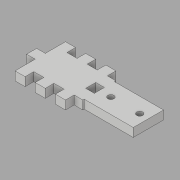
# Autodesk Inventor part: g_arm_v_1
Saved by Autodesk Inventor 2019 (Build 230136000, 136)
## iProperties
Created: 2021-11-02
Part Number: g_arm_v_1
Material: Generic
Document SubType Name: Modeling
Designer: Mohamed
Density: 1 g/cm^3
Appearance: Default
Author: Mohamed
Autodesk Inventor part; units mm, degrees
ref_plane "YZ Plane" through (0, 0, 0) normal (1, 0, 0) x (0, 1, 0)
ref_plane "XZ Plane" through (0, 0, 0) normal (0, 1, 0) x (-1, 0, 0)
ref_plane "XY Plane" through (0, 0, 0) normal (0, 0, 1) x (1, 0, 0)
sketch "Sketch1" plane through (0, 0, 0) normal (1, 0, 0) x (0, 1, 0)
  point P0 (0, 0)
sketch "Sketch2" plane through (0, 0, 0) normal (0, 1, 0) x (-1, 0, 0)
  line L0 (0, 0) -> (35, 0)
  line L1 (35, -21) -> (0, -21)
  line L2 (35, -7) -> (41, -7)
  line L3 (41, -7) -> (41, -14)
  line L4 (41, -14) -> (35, -14)
  line L5 (35, 0) -> (35, -7)
  line L6 (35, -14) -> (35, -21)
  line L7 (0, -21) -> (-40, -21)
  line L8 (-40, -21) -> (-40, 0)
  line L9 (-40, 0) -> (0, 0)
  circle A0 centre (-34, -10.5) radius 2.1
  circle A1 centre (-14, -10.5) radius 2.1
  line L10 (0, -7) -> (-6, -7)
  line L11 (-6, -7) -> (-6, -14)
  line L12 (-6, -14) -> (0, -14)
  line L13 (0, -14) -> (0, -7)
  dimension "d0" = 35
  dimension "d1" = 21
  dimension "d2" = 7
  dimension "d3" = 6
  dimension "d4" = 7
  dimension "d5" = 40
  dimension "d8" = 4.2
  dimension "d10" = 4.2
  dimension "d11" = 6
  dimension "d12" = 7
  constraints: 28 end point, 6 perpendicular, 3 horizontal, 2 centre point, 2 vertical, 1 parallel
  measures "d0" distance of L1.start L1.end
  measures "d1" distance of L0.end L1.start
  measures "d2" distance of L0.end L2.start
  measures "d3" distance of L2.start L2.end
  measures "d4" distance of L2.end L3.end
  measures "d5" distance of L1.end L7.end
  measures "d8" diameter of A0
  measures "d10" diameter of A1
  measures "d11" distance of L10.start L10.end
  measures "d12" distance of L10.end L11.end
extrude "Extrusion1" add sketch "Sketch2" along normal blind 6
sketch "Sketch3" plane through (0, 6, 0) normal (0, 1, 0) x (1, 0, 0)
  line L0 (0, -1) -> (-35, -1)
  line L1 (-35, 0) -> (40, 0) projected
  line L2 (-35, -1) -> (-35, 0)
  line L3 (-35, 21) -> (-35, 14) projected
  line L4 (-35, 21) -> (6, 21)
  line L5 (6, 21) -> (6, 22)
  line L6 (6, 22) -> (-35, 22)
  line L7 (-35, 22) -> (-35, 21)
  line L8 (0, -1) -> (6, -1)
  line L9 (6, -1) -> (6, 0)
  point P0 (0, 0)
  dimension "d15" = 1
  dimension "d17" = 41
  dimension "d18" = 1
  dimension "d21" = 6
  constraints: 16 end point, 3 perpendicular, 2 horizontal, 2 parallel, 1 point on line
  measures "d15" distance of point (0, 0) L0.start
  measures "d17" distance of L6.end L5.end
  measures "d18" distance of L5.end L4.end
  measures "d21" distance of L0.start L8.end
extrude "Extrusion2" add sketch "Sketch3" against normal blind 6
sketch "Sketch4" plane through (0, 6, 0) normal (0, 1, 0) x (1, 0, 0)
  line L0 (6, -1) -> (-35, -1) projected
  line L1 (0, -1) -> (-7, -1)
  line L2 (-7, -1) -> (-7, -7)
  line L3 (-7, -7) -> (0, -7)
  line L4 (0, -7) -> (0, -1)
  line L5 (6, 22) -> (-35, 22) projected
  line L6 (0, 22) -> (-7, 22)
  line L7 (-7, 22) -> (-7, 28)
  line L8 (-7, 28) -> (0, 28)
  line L9 (0, 28) -> (0, 22)
  point P0 (0, 0)
  dimension "d22" = 7
  dimension "d23" = 6
  dimension "d24" = 7
  dimension "d25" = 6
  constraints: 16 end point, 4 parallel, 2 horizontal, 2 perpendicular, 2 point on line
  measures "d22" distance of L3.end L2.end
  measures "d23" distance of L2.end L1.end
  measures "d24" distance of L7.end L8.end
  measures "d25" distance of L6.end L7.end
extrude "Extrusion3" add sketch "Sketch4" against normal blind 6
pattern_linear "Rectangular Pattern1" count 3 spacing 14 along (-1, 0, 0) of "Extrusion3"
body "Solid1"
